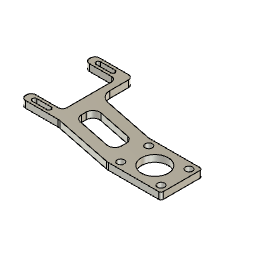
mount-brake (Autodesk Fusion 360 design; units mm, degrees)
Autodesk Fusion 360 part; units mm, degrees
sketch "Sketch24" plane through (0, 0, 0) normal (0, 0, 1) x (1, 0, 0)
  line L0 (0, 0) -> (24, 0)
  line L1 (24, 0) -> (24, 18.5)
  line L2 (24, 18.5) -> (0, 18.5)
  line L3 (0, 18.5) -> (0, 0)
  dimension "d200" = 24
  dimension "d201" = 18.5
  constraint horizontal L0
  constraint vertical L1
  constraint horizontal L2
  constraint vertical L3
  constraint coincident L0.start L3.end
  measures "d200" distance of L0.start L0.end
  measures "d201" distance of L0.start L2.end
sketch "Sketch25" plane through (0, 0, 0) normal (0, 0, 1) x (1, 0, 0)
  line L0 (0, 0) -> (24, 0)
  line L1 (0, 18.5) -> (0, 0)
extrude "Extrude16" add sketch "Sketch24" along normal blind 3
sketch "Sketch26" plane through (0, 0, 3) normal (0, 0, 1) x (-1, 0, 0)
  line L0 (0, -18.5) -> (0, 0)
  line L1 (0, 0) -> (-24, 0)
  line L2 (-24, 0) -> (-24, -18.5)
  line L3 (-24, -18.5) -> (0, -18.5)
  point P0 (-3, -3)
  dimension "d206" = 3
  dimension "d207" = 3
  measures "d206" distance of L0 P0
  measures "d207" distance of L1 P0
hole "Hole7" at (3, 3, 3) direction (0, 0, -1) diameter 3.2 depth 3 tip angle 118
pattern_linear "R-Pattern3" count 2 spacing 18 along (1, 0, 0) count 2 spacing 12.5 along (0, 1, 0) of "Hole7"
sketch "Sketch27" plane through (0, 0, 0) normal (0, 0, 1) x (1, 0, 0)
  line L0 (-44, 10) -> (-30, 10)
  line L1 (-30, 10) -> (-30, 34)
  line L2 (-30, 34) -> (-44, 34)
  line L3 (-44, 34) -> (-44, 10) construction
  line L4 (-41.25, 37.25) -> (-32.75, 37.25)
  line L5 (-32.75, 37.25) -> (-32.75, 35.25)
  line L6 (-32.75, 35.25) -> (-41.25, 35.25)
  line L7 (-41.25, 35.25) -> (-41.25, 37.25)
  line L8 (-41.25, 8.75) -> (-32.75, 8.75)
  line L9 (-32.75, 8.75) -> (-32.75, 6.75)
  line L10 (-32.75, 6.75) -> (-41.25, 6.75)
  line L11 (-41.25, 6.75) -> (-41.25, 8.75)
  line L12 (-44, 34) -> (-44, 38.5)
  line L13 (-44, 38.5) -> (-27, 38.5)
  line L14 (-44, 10) -> (-44, 5.5)
  line L15 (-44, 5.5) -> (-27, 5.5)
  line L16 (-27, 5.5) -> (0, 0)
  line L17 (0, 0) -> (0, 18.5)
  line L18 (0, 18.5) -> (-27, 24)
  line L19 (-27, 24) -> (-27, 5.5) construction
  line L20 (-27, 38.5) -> (-27, 24)
  line L21 (-24, 18.2862) -> (-3, 14.0084)
  line L22 (-3, 14.0084) -> (-3, 5.7138)
  line L23 (-3, 5.7138) -> (-24, 9.9916)
  line L24 (-24, 9.9916) -> (-24, 18.2862)
  dimension "d215" = 14
  dimension "d216" = 24
  dimension "d217" = 30
  dimension "d218" = 10
  dimension "d219" = 8.5
  dimension "d220" = 2
  dimension "d221" = 2.75
  dimension "d222" = 1.25
  dimension "d223" = 8.5
  dimension "d224" = 2
  dimension "d225" = 2.75
  dimension "d226" = 1.25
  dimension "d227" = 4.5
  dimension "d228" = 17
  dimension "d229" = 4.5
  dimension "d230" = 17
  dimension "d231" = 18.5
  dimension "d232" = 3
  dimension "d233" = 3
  dimension "d235" = 5
  dimension "d236" = 5
  constraint horizontal L0
  constraint vertical L1
  constraint horizontal L2
  constraint vertical L3
  constraint horizontal L4
  constraint vertical L5
  constraint horizontal L6
  constraint vertical L7
  constraint horizontal L8
  constraint vertical L9
  constraint horizontal L10
  constraint vertical L11
  constraint perpendicular L2 L12
  constraint perpendicular L12 L13
  constraint perpendicular L0 L14
  constraint perpendicular L14 L15
  constraint coincident L16.end L17.start
  constraint vertical L17
  constraint parallel L16 L18
  constraint vertical L19
  constraint parallel L18 L21
  constraint parallel L21 L23
  measures "d215" distance of L0.start L0.end
  measures "d216" distance of L0.start L2.end
  measures "d217" horizontal distance of L16.end L0.end
  measures "d218" vertical distance of L16.end L0.end
  measures "d219" distance of L4.start L4.end
  measures "d220" distance of L4.start L6.end
  measures "d221" distance of L2.end L7
  measures "d222" distance of L2 L6
  measures "d223" distance of L8.start L8.end
  measures "d224" distance of L8.start L10.end
  measures "d225" distance of L0.start L11
  measures "d226" distance of L0 L8
  measures "d227" distance of L2.end L12.end
  measures "d228" distance of L12.end L13.end
  measures "d229" distance of L0.start L14.end
  measures "d230" distance of L14.end L15.end
  measures "d231" distance of L16.end L17.end
  measures "d232" distance of L19 L24
  measures "d233" distance of L17 L22
  measures "d235" distance of L18 L21
  measures "d236" distance of L16 L23
extrude "Extrude17" add sketch "Sketch27" along normal blind 3
fillet "Fillet20" radius 1 2 edges at (24, 0, 1.5) (24, 18.5, 1.5)
fillet "Fillet21" radius 3 4 edges at (-24, 18.2862, 1.5) (-3, 14.0084, 1.5) (-3, 5.7138, 1.5) (-24, 9.9916, 1.5)
fillet "Fillet22" radius 5 4 edges at (0, 18.5, 1.5) (0, 0, 1.5) (-27, 5.5, 1.5) (-27, 24, 1.5)
fillet "Fillet23" radius 2 7 edges at (-44, 38.5, 1.5) (-44, 34, 1.5) (-44, 10, 1.5) (-44, 5.5, 1.5) (-27, 38.5, 1.5) (-30, 34, 1.5) (-30, 10, 1.5)
fillet "Fillet24" radius 1 8 edges at (-32.75, 37.25, 1.5) (-32.75, 35.25, 1.5) (-41.25, 35.25, 1.5) (-41.25, 37.25, 1.5) (-41.25, 8.75, 1.5) (-41.25, 6.75, 1.5) (-32.75, 6.75, 1.5) (-32.75, 8.75, 1.5)
sketch "Sketch28" plane through (0, 0, 3) normal (0, 0, 1) x (-1, 0, 0)
  arc A0 (27, -36.5) -> (29, -38.5) centre (29, -36.5) ccw
  line L0 (29, -38.5) -> (42, -38.5)
  arc A1 (42, -38.5) -> (44, -36.5) centre (42, -36.5) ccw
  line L1 (44, -36.5) -> (44, -36)
  arc A2 (44, -36) -> (42, -34) centre (42, -36) ccw
  line L2 (42, -34) -> (32, -34)
  arc A3 (30, -32) -> (32, -34) centre (32, -32) ccw
  line L3 (30, -32) -> (30, -12)
  arc A4 (32, -10) -> (30, -12) centre (32, -12) ccw
  line L4 (32, -10) -> (42, -10)
  arc A5 (42, -10) -> (44, -8) centre (42, -8) ccw
  line L5 (44, -8) -> (44, -7.5)
  arc A6 (44, -7.5) -> (42, -5.5) centre (42, -7.5) ccw
  line L6 (42, -5.5) -> (27.5041, -5.5)
  arc A7 (26.5061, -5.3994) -> (27.5041, -5.5) centre (27.5041, -0.5) ccw
  line L7 (26.5061, -5.3994) -> (0.4939, -0.1006)
  arc A8 (0.4939, -0.1006) -> (-0.5041, 0) centre (-0.5041, -5) ccw
  line L8 (-0.5041, 0) -> (-23, 0)
  arc A9 (-23, 0) -> (-24, -1) centre (-23, -1) ccw
  line L9 (-24, -1) -> (-24, -17.5)
  arc A10 (-24, -17.5) -> (-23, -18.5) centre (-23, -17.5) ccw
  line L10 (-23, -18.5) -> (-0.5041, -18.5)
  arc A11 (0.4939, -18.6006) -> (-0.5041, -18.5) centre (-0.5041, -23.5) ccw
  line L11 (0.4939, -18.6006) -> (22.998, -23.1848)
  arc A12 (27, -28.0842) -> (22.998, -23.1848) centre (22, -28.0842) ccw
  line L12 (27, -28.0842) -> (27, -36.5)
  line L13 (33.75, -6.75) -> (40.25, -6.75)
  arc A13 (40.25, -8.75) -> (40.25, -6.75) centre (40.25, -7.75) ccw
  line L14 (40.25, -8.75) -> (33.75, -8.75)
  arc A14 (33.75, -6.75) -> (33.75, -8.75) centre (33.75, -7.75) ccw
  line L15 (6.5988, -6.4469) -> (21.5988, -9.5024)
  arc A15 (24, -12.4421) -> (21.5988, -9.5024) centre (21, -12.4421) ccw
  line L16 (24, -12.4421) -> (24, -14.6135)
  arc A16 (20.4012, -17.5531) -> (24, -14.6135) centre (21, -14.6135) ccw
  line L17 (20.4012, -17.5531) -> (5.4012, -14.4976)
  arc A17 (3, -11.5579) -> (5.4012, -14.4976) centre (6, -11.5579) ccw
  line L18 (3, -11.5579) -> (3, -9.3865)
  arc A18 (6.5988, -6.4469) -> (3, -9.3865) centre (6, -9.3865) ccw
  line L19 (33.75, -35.25) -> (40.25, -35.25)
  arc A19 (41.25, -36.25) -> (40.25, -35.25) centre (40.25, -36.25) ccw
  arc A20 (40.25, -37.25) -> (41.25, -36.25) centre (40.25, -36.25) ccw
  line L20 (40.25, -37.25) -> (33.75, -37.25)
  arc A21 (32.75, -36.25) -> (33.75, -37.25) centre (33.75, -36.25) ccw
  arc A22 (33.75, -35.25) -> (32.75, -36.25) centre (33.75, -36.25) ccw
  circle A23 centre (-21, -15.5) radius 1.6
  circle A24 centre (-3, -15.5) radius 1.6
  circle A25 centre (-21, -3) radius 1.6
  circle A26 centre (-3, -3) radius 1.6
  circle A27 centre (-12, -9.25) radius 6
  point P0 (-12, -9.25)
  dimension "d249" = 12
  dimension "d250" = 9.25
  dimension "d251" = 12
  constraint coincident P0 A27.centre
  measures "d249" horizontal distance of origin A27.centre
  measures "d250" vertical distance of origin A27.centre
  measures "d251" diameter of A27
extrude "Extrude18" cut sketch "Sketch28" against normal blind 3 contours A27
equation "d250 = ( 18.5 / 2 ) * 1 mm"
